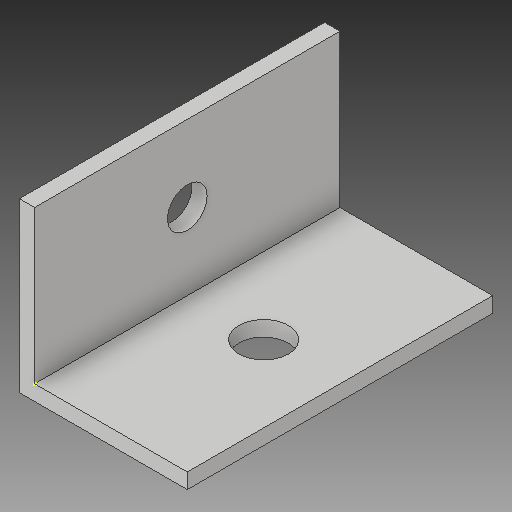
# Autodesk Inventor part: Bed Plate Support
Saved by Autodesk Inventor 2018 (Build 220112000, 112)
## iProperties
Created: 2017-04-14
Part Number: Bed Plate Support
Material: Generic
Document SubType Name: Modeling
Designer: Administrator
Density: 1 g/cm^3
Appearance: Default
Author: Administrator
Autodesk Inventor part; units mm, degrees
ref_plane "YZ Plane" through (0, 0, 0) normal (1, 0, 0) x (0, 1, 0)
ref_plane "XZ Plane" through (0, 0, 0) normal (0, 1, 0) x (-1, 0, 0)
ref_plane "XY Plane" through (0, 0, 0) normal (0, 0, 1) x (1, 0, 0)
sketch "Sketch1" plane through (0, 0, 0) normal (0, 0, 1) x (1, 0, 0)
  point P0 (0, 0)
sketch "Sketch2" plane through (0, 0, 0) normal (0, 0, 1) x (1, 0, 0)
  line L0 (0, 0) -> (0, 20)
  line L1 (0, 20) -> (-2, 20)
  line L2 (-2, 20) -> (-2, -2)
  line L3 (-2, -2) -> (20, -2)
  line L4 (20, -2) -> (20, 0)
  line L5 (20, 0) -> (0, 0)
  dimension "d0" = 20
  dimension "d1" = 2
  dimension "d2" = 22
  dimension "d3" = 22
  dimension "d4" = 2
  dimension "d5" = 20
  constraints: 12 end point, 4 perpendicular, 1 vertical
  measures "d0" distance of L0.start L0.end
  measures "d1" distance of L0.end L1.end
  measures "d2" distance of L1.end L2.end
  measures "d3" distance of L2.end L3.end
  measures "d4" distance of L3.end L4.end
  measures "d5" distance of L4.end L0.start
extrude "Extrusion1" add sketch "Sketch2" against normal blind 40
sketch "Sketch3" plane through (0, 0, 0) normal (0, 1, 0) x (1, 0, 0)
  point P0 (0, 0)
sketch "Sketch4" plane through (0, 0, 0) normal (0, 1, 0) x (1, 0, 0)
  circle A0 centre (10, 20) radius 3.25
  point P0 (0, 0)
  dimension "d9" = 6.5
  constraints: 1 centre point
  measures "d9" diameter of A0
hole "Hole1" at (10, 0, -20) direction (0, -1, 0) diameter 6.5 end through all
sketch "Sketch5" plane through (0, 0, 0) normal (1, 0, 0) x (0, 0, -1)
  circle A0 centre (20, 10) radius 2.6
  point P0 (0, 0)
  dimension "d17" = 5.2
  constraints: 1 centre point
  measures "d17" diameter of A0
hole "Hole2" at (0, 10, -20) direction (-1, 0, 0) diameter 5.2 end through all
body "Solid1"
